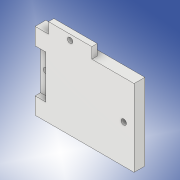
# Autodesk Inventor part: SP003
Saved by Autodesk Inventor 2017 SP1 (Build 210196100, 196)
## iProperties
Created: 2017-08-09
Part Number: SP003
Material: ABS Plastic
Document SubType Name: Modeling
Designer: Zach
Density: 1.06 g/cm^3
Appearance: CR White
Author: Zach
Autodesk Inventor part; units mm, degrees
ref_plane "YZ Plane" through (0, 0, 0) normal (1, 0, 0) x (0, 1, 0)
ref_plane "XZ Plane" through (0, 0, 0) normal (0, 1, 0) x (-1, 0, 0)
ref_plane "XY Plane" through (0, 0, 0) normal (0, 0, 1) x (1, 0, 0)
sketch "Sketch1" plane through (0, 0, 0) normal (0, 0, 1) x (1, 0, 0)
  line L0 (0, 0) -> (72.4, 0)
  line L1 (72.4, 0) -> (72.4, 71)
  line L2 (72.4, 71) -> (0, 71)
  line L3 (0, 71) -> (0, 0)
  dimension "d0" = 72.4
  dimension "d1" = 71
  constraints: 8 end point, 2 parallel, 1 horizontal, 1 perpendicular
  measures "d0" distance of L1.end L2.end
  measures "d1" distance of L0.end L1.end
extrude "Extrusion1" add sketch "Sketch1" along normal blind 10
sketch "Sketch2" plane through (0, 0, 10) normal (0, 0, 1) x (1, 0, 0)
  line L0 (12.4, 71) -> (52.4, 71)
  line L1 (52.4, 71) -> (52.4, 81)
  line L2 (52.4, 81) -> (12.4, 81)
  line L3 (12.4, 81) -> (12.4, 71)
  line L4 (72.4, 0) -> (72.4, 71) projected
  line L5 (72.4, 71) -> (0, 71) projected
  circle A0 centre (32.4, 76) radius 2.5
  point P0 (0, 0)
  point P1 (36.2, 71)
  point P2 (52.4, 76)
  point P3 (32.4, 81)
  dimension "d4" = 40
  dimension "d5" = 10
  dimension "d6" = 20
  dimension "d7" = 5
  constraints: 8 end point, 3 midpoint, 2 parallel, 1 centre point, 1 horizontal, 1 horizontal alignment, 1 perpendicular, 1 point on line, 1 vertical alignment
  measures "d4" distance of L2.end L1.end
  measures "d5" distance of L1.end L0.end
  measures "d6" distance between parallel lines of L4 L1
  measures "d7" diameter of A0
extrude "Extrusion2" add sketch "Sketch2" against normal blind 5
sketch "Sketch3" plane through (0, 0, 10) normal (0, 0, 1) x (1, 0, 0)
  line L0 (72.4, 0) -> (72.4, 71) projected
  line L1 (72.4, 0) -> (91.4, 0)
  line L2 (91.4, 0) -> (91.4, 71)
  line L3 (91.4, 71) -> (72.4, 71)
  line L4 (72.4, 71) -> (72.4, 0)
  line L5 (72.4, 71) -> (52.4, 71) projected
  point P0 (0, 0)
  dimension "d10" = 19
  constraints: 8 end point, 2 parallel, 1 coincident, 1 horizontal, 1 perpendicular
  measures "d10" distance of L3.end L2.end
extrude "Extrusion3" add sketch "Sketch3" against normal blind 10
sketch "Sketch4" plane through (0, 0, 10) normal (0, 0, 1) x (1, 0, 0)
  circle A0 centre (81.9, 35.5) radius 2.5
  line L0 (91.4, 0) -> (91.4, 71) projected
  line L1 (91.4, 35.5) -> (72.4, 35.5) construction
  point P0 (0, 0)
  point P1 (81.9, 62)
  dimension "d15" = 5
  dimension "d31" = 19
  constraints: 2 end point, 2 midpoint, 1 centre point, 1 coincident, 1 horizontal, 1 horizontal alignment, 1 vertical alignment
  measures "d15" diameter of A0
  measures "d31" distance of L1.start L1.end
extrude "Extrusion4" cut sketch "Sketch4" against normal through all
sketch "Sketch5" plane through (0, 0, 10) normal (0, 0, 1) x (1, 0, 0)
  line L0 (0, 0) -> (91.4, 0) projected
  line L1 (12.4, 0) -> (52.4, 0)
  line L2 (52.4, 0) -> (52.4, 10)
  line L3 (52.4, 10) -> (12.4, 10)
  line L4 (12.4, 10) -> (12.4, 0)
  line L5 (0, 71) -> (0, 0) projected
  line L6 (0, 55.5) -> (10, 55.5)
  line L7 (10, 55.5) -> (10, 15.5)
  line L8 (10, 15.5) -> (0, 15.5)
  line L9 (0, 15.5) -> (0, 55.5)
  point P0 (52.4, 81)
  point P1 (12.4, 81)
  point P2 (0, 35.5)
  point P3 (0, 35.5)
  dimension "d22" = 10
  dimension "d25" = 10
  dimension "d26" = 40
  constraints: 16 end point, 4 parallel, 2 horizontal, 2 midpoint, 2 perpendicular, 2 point on line, 2 vertical alignment, 1 coincident
  measures "d22" distance of L2.end L1.end
  measures "d25" distance of L7.end L8.end
  measures "d26" distance of L6.end L7.end
extrude "Extrusion5" cut sketch "Sketch5" against normal blind 5 contours L5 L6 L7 L8
sketch "Sketch6" plane through (0, 0, 5) normal (0, 0, 1) x (1, 0, 0)
  line L0 (0, 15.5) -> (0, 55.5) projected
  line L1 (10, 15.5) -> (0, 15.5) projected
  line L2 (10, 55.5) -> (10, 15.5) projected
  line L3 (0, 55.5) -> (10, 55.5) projected
  line L4 (52.4, 0) -> (12.4, 0) projected
  line L5 (52.4, 10) -> (52.4, 0) projected
  line L6 (12.4, 10) -> (52.4, 10) projected
  line L7 (12.4, 0) -> (12.4, 10) projected
  circle A0 centre (5, 35.5) radius 2.5
  circle A1 centre (32.4, 5) radius 2.5
  point P0 (0, 0)
  point P1 (0, 35.5)
  point P2 (12.4, 5)
  point P3 (32.4, 10)
  point P4 (5, 55.5)
  dimension "d27" = 5
  dimension "d28" = 5
  constraints: 4 midpoint, 2 centre point, 2 horizontal alignment, 2 vertical alignment
  measures "d27" diameter of A0
  measures "d28" diameter of A1
extrude "Extrusion6" cut sketch "Sketch6" against normal through all contours A0
body "Solid1"
